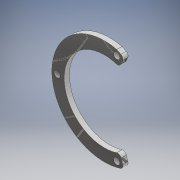
# Autodesk Inventor part: reverse gear reverse lever ring
Saved by Autodesk Inventor 2017 (Build 210142000, 142)
## iProperties
Created: 2018-11-05
Part Number: reverse gear reverse lever ring
Material: Generic
Document SubType Name: Modeling
Designer: User
Density: 1 g/cm^3
Appearance: Default
Author: User
Autodesk Inventor part; units mm, degrees
ref_plane "YZ Plane" through (0, 0, 0) normal (1, 0, 0) x (0, 1, 0)
ref_plane "XZ Plane" through (0, 0, 0) normal (0, 1, 0) x (-1, 0, 0)
ref_plane "XY Plane" through (0, 0, 0) normal (0, 0, 1) x (1, 0, 0)
sketch "Sketch1" plane through (0, 0, 0) normal (0, 1, 0) x (-1, 0, 0)
  arc A0 (-7.2165, -28.9468) -> (-7.2165, 29.397) centre (-0.2165, 0.2251) ccw
  arc A1 (-7.2165, -25.8517) -> (-7.2165, 26.3019) centre (-0.2165, 0.2251) ccw construction
  arc A2 (-7.2165, -21.6838) -> (-7.2165, 22.134) centre (-0.2165, 0.2251) ccw
  line L0 (-7.2165, 33.9307) -> (-7.2165, -32.8883) construction
  circle A3 centre (-7.2165, 26.3019) radius 1.75
  circle A4 centre (-7.2165, -25.8517) radius 1.75
  circle A5 centre (26.7835, 0.2251) radius 1.75
  line L1 (-7.2165, 29.397) -> (-11.2926, 27.3801)
  line L2 (-11.2926, 27.3801) -> (-8.8324, 21.4622)
  line L3 (-8.8324, 21.4622) -> (-7.2165, 22.134)
  line L4 (-7.2165, -28.9468) -> (-11.2102, -27.8268)
  line L5 (-11.2102, -27.8268) -> (-9.1721, -21.092)
  line L6 (-9.1721, -21.092) -> (-7.2165, -21.6838)
  dimension "d14" = 54
  dimension "d16" = 46
  dimension "d17" = 30
  dimension "d19" = 3.5
  dimension "d20" = 3.5
  dimension "d21" = 7
  dimension "d22" = 3.5
  constraints: 14 end point, 7 point on circle, 6 centre point, 4 coincident, 4 point on line, 2 perpendicular, 1 vertical
  measures "d14" diameter of A1
  measures "d16" diameter of A2
  measures "d17" radius of A0
  measures "d19" diameter of A3
  measures "d20" diameter of A4
  measures "d21" horizontal distance of A0.centre A3.centre
  measures "d22" diameter of A5
extrude "Extrusion1" add sketch "Sketch1" along normal blind 3
fillet "Fillet1" radius 2 4 edges at (11.2926, 1.5, 27.3801) (8.8324, 1.5, 21.4622) (11.2102, 1.5, -27.8268) (9.1721, 1.5, -21.092)
body "Solid1"
